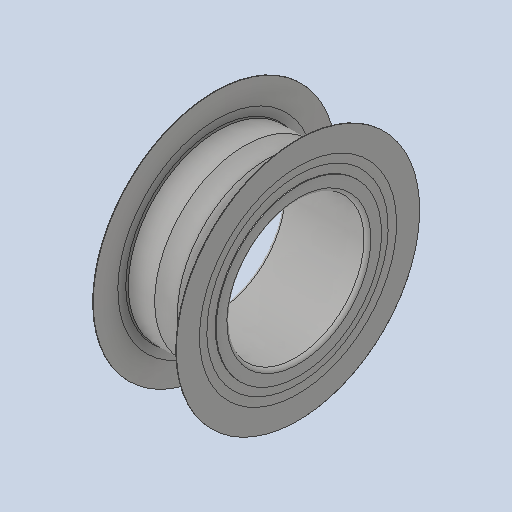
# Autodesk Inventor part: SKF_W 628/8 R-2RS1_PART1
Saved by Autodesk Inventor 2022 (Build 260153000, 153)
## iProperties
Created: 2022-08-03
Part Number: SKF_W 628/8 R-2RS1_PART1
Material: Generic
Catalog Web Link: www.cadenas.de
Description: -Deep groove ball bearings
Vendor: SKF
Document SubType Name: Modeling
Designer: psAdmin
Manufacturer: SKF
Mass: 4 g
Surface Area: 6.95425 cm^2
Volume: 0.180033 cm^3
Density: 1 g/cm^3
Appearance: PSOLRGB-175-175-175
Category: PARTsolutions
Company: SKF
PSOL_IDENT_0: {$CADENAS_DATA/23d-libs/skf/bearings_units_and_housings/ball_bearings/deep_groove_ball_bearings/bb1_
PSOL_IDENT_1: 001_101.prj},215 {VTYP=3D},{NB=SKF_W 628/8 R-2RS1_PART1},{LINA=SKF_W 628/8 R-2RS1_PART1},{NN=BB1_001
PSOL_IDENT_2: _101_PART1},{NOPRJ=TRUE},{DATE=29.07.2022 12:16:16},{GEOMDATE=04.07.2022 10:54:51},{VERSION=},{LINEI
PSOL_IDENT_3: D=22660},{WBVAR=},{WBNUMERIC=}  {NB=SKF_W 628/8 R-2RS1_PART1},{LINA=SKF_W 628/8 R-2RS1_PART1},{KT=DU
PSOL_IDENT_4: MMY},{DESIGNATION=W 628/8 R-2RS1},{R12=0.20},{DD=8.000},{D=16.000},{B=5.000},{C=},{CX=},{CXX=1.1},{C
PSOL_IDENT_5: A=1.100},{XXVARIANT=Flanged outer ring},{XXDESIGN=Single row stainless steel},{XXSEALING=Contact sea
PSOL_IDENT_6: l on both sides},{DESIGN=dgbbwr2zs},{DESIGNIR=dgbbwr2zs},{VARIANT=Flanged outer ring},{DD1=10.50},{D
PSOL_IDENT_7: D2=9.65},{DD2X=},{DD2A=9.65},{D1=13.50},{D1X=0.00},{D2=14.2},{D2A=14.20},{D3=18},{D3X=},{D3A=18.000}
PSOL_IDENT_8: ,{D4=},{HH=0.000},{BB=0.000},{BBX=},{BBA=0.000},{FF=},{R0MAX=0.000},{R0=0.000},{PITCH=12.00},{DW=2.0
PSOL_IDENT_9: 00},{DDAMIN=9.500},{DDAMAX=9.600},{DDBMIN=0.000},{DDBMAX=0.000},{DBMIN=0.000},{DAMAX=0.000},{BBAMIN=
PSOL_IDENT_10: 0.000},{CAMAX=0.000},{RAMAX=0.200},{LOAD1=0.715},{LOAD2=0.300},{LOAD3=0.012},{SPEED1=0},{SPEED2=2600
PSOL_IDENT_11: 0},{KR=0.020},{F0=7.500},{Z=10},{II=1},{MASS=0.004},{BEARING=W 628/8 R-2RS1},{RING=},{HELP=1.250},{H
PSOL_IDENT_12: ELP2=0.900},{DD1ALG=5.250},{YALG=5.250},{PITCH1=12.000},{DW1=2.000},{YALG1=6.750},{HALG1=1.250},{SH=
PSOL_IDENT_13: 4.825},{CU=0.600},{HALG=1.25},{B1=-2.55},{SHIELDHELP=2},{D4A=0.000},{FFA=0.000},{RS1=},{HELP3=0}
NB: SKF_W 628/8 R-2RS1_PART1
NT: Deep groove ball bearings
NBSYN: SKF_$DESIGNATION._PART1
LINA: SKF_W 628/8 R-2RS1_PART1
CATALOG: SKF
DESIGNATION: W 628/8 R-2RS1
R12: 0.2
DD: 8
D: 16
B: 5
XXVARIANT: Flanged outer ring
XXDESIGN: Single row stainless steel
XXSEALING: Contact seal on both sides
DD2: 9.65
D2: 14.2
LOAD1: 0.715
LOAD2: 0.3
LOAD3: 0.012
SPEED1: 0
SPEED2: 26000
BEARING: W 628/8 R-2RS1
SUPPLIER: SKF
ARTICLENO: SKF_W 628/8 R-2RS1_PART1
BOMINFO: SKF_W 628/8 R-2RS1_PART1
CREATOR: CADENAS GmbH
Title: SKF_W 628/8 R-2RS1_PART1
Author: Cadenas PARTsolutions
Comments: Deep groove ball bearings
Autodesk Inventor part; units mm, degrees
ref_plane "YZ Plane" through (0, 0, 0) normal (1, 0, 0) x (0, 1, 0)
ref_plane "XZ Plane" through (0, 0, 0) normal (0, 1, 0) x (-1, 0, 0)
ref_plane "XY Plane" through (0, 0, 0) normal (0, 0, 1) x (1, 0, 0)
sketch "Sketch_40" plane through (0, 0, 0) normal (0, 0, 1) x (1, 0, 0)
  line L0 (2.5, 0) -> (-2.5, 0)
  line L1 (0, 5.2) -> (0, 4.2)
  arc A0 (0, 4.2) -> (0.2, 4) centre (0.2, 4.2) ccw
  line L2 (0.2, 4) -> (4.8, 4)
  arc A1 (4.8, 4) -> (5, 4.2) centre (4.8, 4.2) ccw
  line L3 (5, 4.2) -> (5, 5.2)
  arc A2 (5, 5.2) -> (4.95, 5.25) centre (4.95, 5.2) ccw
  line L4 (4.95, 5.25) -> (3.1614, 5.25)
  arc A3 (1.8386, 5.25) -> (3.1614, 5.25) centre (2.5, 6) ccw
  line L5 (1.8386, 5.25) -> (0.05, 5.25)
  arc A4 (0.05, 5.25) -> (0, 5.2) centre (0.05, 5.2) ccw
  constraints: 12 end point, 10 point on circle, 5 centre point
revolve "Revolution1" add sketch "Sketch_40" angle 360 about axis through (2.5, 0, 0) along (1, 0, 0)
sketch "Sketch_42" plane through (0, 0, 0) normal (0, 0, 1) x (1, 0, 0)
  line L0 (2.5, 0) -> (-2.5, 0)
  line L1 (0, 10.825) -> (0, 4.825)
  line L2 (0, 4.825) -> (0.1, 4.825)
  arc A0 (0.1, 4.825) -> (0.3, 5.025) centre (0.1, 5.025) ccw
  line L3 (0.3, 5.025) -> (0.3, 10.625)
  line L4 (0.3, 10.625) -> (4.7, 10.625)
  line L5 (4.7, 10.625) -> (4.7, 5.025)
  arc A1 (4.7, 5.025) -> (4.9, 4.825) centre (4.9, 5.025) ccw
  line L6 (4.9, 4.825) -> (5, 4.825)
  line L7 (5, 4.825) -> (5, 10.825)
  line L8 (5, 10.825) -> (0, 10.825)
  constraints: 18 end point, 4 point on circle, 2 centre point
revolve "Revolution2" cut sketch "Sketch_42" angle 360 about axis through (2.5, 0, 0) along (1, 0, 0)
sketch "Sketch_44" plane through (0, 0, 0) normal (0, 0, 1) x (1, 0, 0)
  line L0 (5, 0) -> (-5, 0)
  line L1 (4.83, 5.2875) -> (4.89, 4.825)
  line L2 (4.89, 4.825) -> (4.95, 4.825)
  line L3 (4.95, 4.825) -> (4.92, 5.2875)
  line L4 (4.92, 5.2875) -> (4.95, 5.75)
  line L5 (4.95, 5.75) -> (4.95, 7.1)
  line L6 (4.95, 7.1) -> (4.9176, 7.1)
  line L7 (4.9176, 7.1) -> (4.83, 5.75)
  line L8 (4.83, 5.75) -> (4.83, 5.2875)
  constraints: 18 end point
revolve "Revolution3" add sketch "Sketch_44" angle 360 about axis through (5, 0, 0) along (1, 0, 0)
sketch "Sketch_49" plane through (0, 0, 0) normal (0, 0, 1) x (1, 0, 0)
  line L0 (5, 0) -> (-5, 0)
  line L1 (0.07, 4.825) -> (0.13, 4.825)
  line L2 (0.13, 4.825) -> (0.19, 5.2875)
  line L3 (0.19, 5.2875) -> (0.19, 5.75)
  line L4 (0.19, 5.75) -> (0.1024, 7.1)
  line L5 (0.1024, 7.1) -> (0.07, 7.1)
  line L6 (0.07, 7.1) -> (0.07, 5.75)
  line L7 (0.07, 5.75) -> (0.1, 5.2875)
  line L8 (0.1, 5.2875) -> (0.07, 4.825)
  constraints: 18 end point
revolve "Revolution4" add sketch "Sketch_49" angle 360 about axis through (5, 0, 0) along (1, 0, 0)
body "Solid1"
